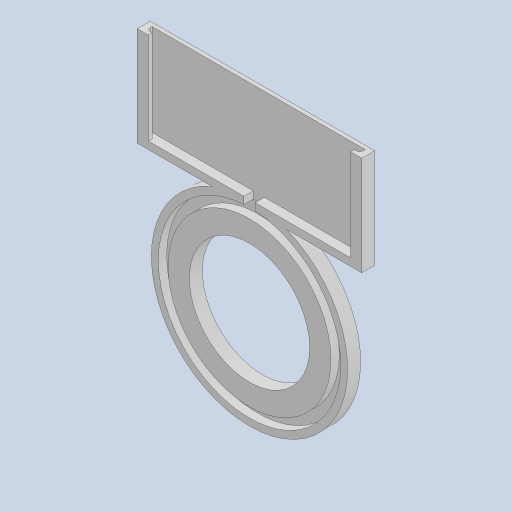
# Autodesk Inventor part: RFID_holder_04
Saved by Autodesk Inventor 2024.4 (Build 284460000, 460)
## iProperties
Created: 2026-03-24
Part Number: RFID_holder_04
Material: Generic
Document SubType Name: Modeling
Designer: Admin
Density: 1 g/cm^3
Appearance: Default
Author: Admin
Autodesk Inventor part; units mm, degrees
ref_plane "YZ Plane" through (0, 0, 0) normal (1, 0, 0) x (0, 1, 0)
ref_plane "XZ Plane" through (0, 0, 0) normal (0, 1, 0) x (-1, 0, 0)
ref_plane "XY Plane" through (0, 0, 0) normal (0, 0, 1) x (1, 0, 0)
derived "PCB.ipt"
sketch "Sketch1: PCB" plane through (0, 0, 0) normal (0, 0, 1) x (1, 0, 0)
  line L0 (-22.0554, 53.3935) -> (34.5446, 53.3935)
  line L1 (34.5446, 53.3935) -> (34.5446, 28.5935)
  line L2 (34.5446, 28.5935) -> (-22.0554, 28.5935)
  line L3 (-22.0554, 28.5935) -> (-22.0554, 53.3935)
  line L4 (2.3446, 55.1935) -> (9.9446, 55.1935)
  line L5 (9.9446, 55.1935) -> (9.9446, 45.9935)
  line L6 (9.9446, 45.9935) -> (2.3446, 45.9935)
  line L7 (2.3446, 45.9935) -> (2.3446, 55.1935)
  point P0 (0, 0)
sketch "Sketch3: PCB base & outside walls" plane through (0, 0, 0) normal (0, 0, 1) x (1, 0, 0)
  line L0 (-22.0554, 28.5935) -> (-22.0554, 53.3935) construction
  line L1 (-22.0554, 53.3935) -> (34.5446, 53.3935) construction
  line L2 (34.5446, 28.5935) -> (-22.0554, 28.5935) construction
  line L3 (34.5446, 53.3935) -> (34.5446, 28.5935) construction
  line L4 (-24.0554, 53.3935) -> (36.5446, 53.3935)
  line L5 (36.5446, 53.3935) -> (36.5446, 26.5935)
  line L6 (36.5446, 26.5935) -> (-24.0554, 26.5935)
  line L7 (-24.0554, 26.5935) -> (-24.0554, 53.3935)
  line L8 (35.0446, 53.3935) -> (35.0446, 28.5935)
  line L9 (35.0446, 28.5935) -> (-22.5554, 28.5935)
  line L10 (-22.5554, 28.5935) -> (-22.5554, 53.3935)
  point P0 (0, 0)
  dimension "d28" = 2
  dimension "d31" = 0.5
  dimension "d32" = 0.5
  dimension "d45" = 1.5
  dimension "d46" = 1.5
  dimension "d53" = 57.6
  constraints: 14 end point, 2 collinear, 2 point on line
  measures "d28" distance between parallel lines of L6 L2
  measures "d31" distance between parallel lines of L0 L10
  measures "d32" distance between parallel lines of L8 L3
  measures "d45" distance between parallel lines of L10 L7
  measures "d46" distance between parallel lines of L5 L8
  measures "d53" distance between parallel lines of L8 L10
sketch "Sketch4: PCB slider" plane through (0, 0, 0) normal (0, 0, 1) x (1, 0, 0)
  line L0 (-21.0554, 53.3935) -> (-21.0554, 28.5935)
  line L1 (33.5446, 53.3935) -> (33.5446, 28.5935)
  line L2 (-24.0554, 53.3935) -> (36.5446, 53.3935) projected
  line L3 (35.0446, 28.5935) -> (-22.5554, 28.5935) projected
  line L4 (-22.0554, 28.5935) -> (-22.0554, 53.3935) construction
  line L5 (34.5446, 53.3935) -> (34.5446, 28.5935) construction
  line L6 (35.0446, 53.3935) -> (35.0446, 28.5935) projected
  line L7 (-22.5554, 28.5935) -> (-22.5554, 53.3935) projected
  point P0 (0, 0)
  dimension "d33" = 1
  dimension "d34" = 1
  constraints: 4 end point, 4 point on line
  measures "d33" distance between parallel lines of L0 L4
  measures "d34" distance between parallel lines of L5 L1
extrude "Ex4: PCB base" add sketch "Sketch3: PCB base & outside walls" along normal blind 1
extrude "Ex5: PCB outside walls" add sketch "Sketch3: PCB base & outside walls" along normal blind 3.5 contours L4 L10 L9 L8 L5 L6 L7
extrude "Ex6: PCB slider" add sketch "Sketch4: PCB slider" against normal blind 1 from surface at 3.5 contours L0 L3 L7 L2 | L2 L6 L3 L1
fillet "Fillet1" radius 1 2 edges at (-22.5554, 40.9935, 2.5) (35.0446, 40.9935, 2.5)
sketch "Sketch1: around tube" plane through (0, 0, 0) normal (0, 0, 1) x (1, 0, 0)
  circle A0 centre (6.2446, 2.0935) radius 16.25
  circle A1 centre (6.2446, 2.0935) radius 20.25
  line L0 (36.5446, 26.5935) -> (-24.0554, 26.5935) construction
  circle A2 centre (6.2446, 2.0935) radius 26.5 construction
  circle A3 centre (6.2446, 2.0935) radius 24.75 construction
  line L1 (35.0446, 28.5935) -> (-22.5554, 28.5935) construction
  line L2 (-3.2257, 26.8435) -> (15.7149, 26.8435) construction
  point P0 (0, 0)
  point P1 (6.2446, 26.5935)
  dimension "d0" = 32.5
  dimension "d1" = 4
  dimension "d42" = 53
  dimension "d43" = 49.5
  dimension "d47" = 1.75
  constraints: 4 centre point, 3 coincident, 2 end point, 2 point on circle, 2 tangent, 1 horizontal, 1 midpoint, 1 vertical alignment
  measures "d0" diameter of A0
  measures "d1" radial gap between concentric circles of A1 A0
  measures "d42" diameter of A2
  measures "d43" diameter of A3
  measures "d47" radial gap between concentric circles of A3 A2
sketch "Sketch2: RFID holder" plane through (0, 0, 0) normal (0, 0, 1) x (1, 0, 0)
  circle A0 centre (6.2446, 2.0935) radius 16.25 projected
  circle A1 centre (6.2446, 2.0935) radius 22
  circle A2 centre (6.2446, 2.0935) radius 24.625
  circle A3 centre (6.2446, 2.0935) radius 26.5
  line L0 (4.7446, 28.5935) -> (4.7446, 26.6728)
  line L1 (7.7446, 28.5935) -> (7.7446, 26.6728)
  line L2 (35.0446, 28.5935) -> (-22.5554, 28.5935) projected
  point P0 (0, 0)
  point P1 (7.7446, 28.5511)
  point P2 (4.7446, 28.5511)
  point P3 (6.2446, 28.5935)
  dimension "RFID_coil_ID" = 44
  dimension "RFID_coil_OD" = 49.25
  dimension "d7" = 1.875
  dimension "d48" = 53
  dimension "d49" = 3
  dimension "d50" = 1.5
  constraints: 4 coincident, 4 end point, 3 centre point, 2 point on circle, 2 point on line, 1 perpendicular
  measures "RFID_coil_ID" diameter of A1
  measures "RFID_coil_OD" diameter of A2
  measures "d7" radial gap between concentric circles of A2 A3
  measures "d48" diameter of A3
  measures "d49" distance between parallel lines of L1 L0
  measures "d50" horizontal distance of L0.start A2.centre
extrude "Ex1: around tube" [suppressed]
extrude "Ex2: RFID holder base" add sketch "Sketch2: RFID holder" along normal blind 3.5 contours A1 | A2 | A2 L1 A3 L0 | A2 L0 A3 L1
extrude "Ex3: RFID inset" cut sketch "Sketch2: RFID holder" against normal blind 2.25 from surface at 3.5 contours A2
extrude "Ex4: RFID wire cutout" cut sketch "Sketch2: RFID holder" against normal up to surface (2.5 mm away) from surface at 3.5 contours A2 L0 A3 L1 | A3 L2 L1 | L0 L2 A3 picked at (6.2446, 27.3401)
equation "\"d32\" = d31"
equation "\"d46\" = d45"
equation "\"d50\" = 0.5 * d49"
body "Solid1"
